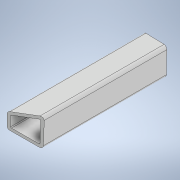
# Autodesk Inventor part: handle_body_final
Saved by Autodesk Inventor 2021 (Build 250183000, 183)
## iProperties
Created: 2021-09-13
Part Number: handle_body_final
Material: Generisch
Document SubType Name: Modeling
Designer: Alexander Claas
Density: 1 g/cm^3
Appearance: Vorgabe
Author: Alexander Claas
Autodesk Inventor part; units mm, degrees
ref_plane "YZ Plane" through (0, 0, 0) normal (1, 0, 0) x (0, 1, 0)
ref_plane "XZ Plane" through (0, 0, 0) normal (0, 1, 0) x (-1, 0, 0)
ref_plane "XY Plane" through (0, 0, 0) normal (0, 0, 1) x (1, 0, 0)
sketch "Skizze1" plane through (0, 0, 0) normal (0, 0, 1) x (1, 0, 0)
  line L0 (25.5223, 16.961) -> (0, 12)
  line L1 (0, 12) -> (0, 0)
  line L2 (0, 0) -> (25.0305, -7.0339)
  line L3 (25.0305, -7.0339) -> (25.5223, 16.961)
  line L4 (-3, 14.473) -> (28.5978, 20.615)
  line L5 (28.5978, 20.615) -> (27.9504, -10.9707)
  line L6 (27.9504, -10.9707) -> (-3, -2.2732)
  line L7 (-3, -2.2732) -> (-3, 14.473)
  dimension "d0" = 26
  dimension "d1" = 12
  dimension "d3" = 26
  dimension "d4" = 24
  dimension "d7" = 101
  dimension "d8" = 77.826
  dimension "d9" = 3
  dimension "d10" = 3
  dimension "d11" = 3
  dimension "d12" = 3
  constraints: 16 end point, 4 parallel, 1 coincident, 1 vertical
  measures "d0" distance of L0.start L0.end
  measures "d1" distance of L0.end L1.end
  measures "d3" distance of L1.end L2.end
  measures "d4" distance of L2.end L0.start
  measures "d7" angle of L1 L0
  measures "d8" angle of L3 L0
  measures "d9" distance between parallel lines of L7 L1
  measures "d10" distance between parallel lines of L4 L0
  measures "d11" distance between parallel lines of L5 L3
  measures "d12" distance between parallel lines of L2 L6
extrude "Extrusion1" add sketch "Skizze1" along normal blind 150
sketch "Skizze3" plane through (0, 0, 0) normal (0, 1, 0) x (-1, 0, 0)
  line L0 (3, 0) -> (3, 150) construction
  line L1 (-27.9504, 0) -> (-28.5978, 0) construction
  line L2 (-28.5978, 0) -> (-28.5978, 150) construction
  line L3 (-27.9504, 150) -> (-28.5978, 150) construction
  line L4 (-27.9504, 0) -> (-27.9504, 150) construction
  line L5 (3, 0) -> (-28.5978, 6.7163)
  line L6 (-28.5978, 6.7163) -> (-28.5978, 0)
  line L7 (3, 150) -> (-28.5978, 140.9395)
  line L8 (-28.5978, 150) -> (-28.5978, 140.9395)
  line L9 (3, 150) -> (-27.9504, 150) projected
  line L10 (-28.5978, 150) -> (3, 150)
  line L11 (-27.9504, 0) -> (-28.5978, 0) projected
  line L12 (-28.5978, 0) -> (3, 0)
  point P0 (0, 0)
  dimension "d19" = 78
  dimension "d20" = 74
  dimension "d25" = 150
  constraints: 12 end point, 3 collinear, 2 point on line, 1 horizontal
  measures "d19" angle of L0 L5
  measures "d20" angle of L0 L7
  measures "d25" distance of L0.start L0.end
extrude "Extrusion2" cut sketch "Skizze3" along normal mid plane 149
fillet "Rundung1" radius 3 4 edges at (-3, -2.2732, 75) (27.9504, -10.9707, 73.8519) (-3, 14.473, 75) (28.5978, 20.615, 73.8279)
fillet "Rundung1" radius 1 4 edges at (25.5223, 16.961, 73.942) (25.0305, -7.0339, 73.9602) (0, 0, 74.8887) (0, 12, 74.8887)
equation "\"d10\" = d9"
equation "\"d11\" = d9"
equation "\"d12\" = d9"
